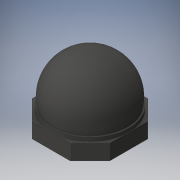
# Autodesk Inventor part: Drone Cover
Saved by Autodesk Inventor 2016 (Build 200138000, 138)
## iProperties
Created: 2015-05-23
Part Number: Drone Cover
Material: Generic
Document SubType Name: Modeling
Designer: Admin
Density: 1 g/cm^3
Appearance: Default
Mass: 29.2837 g
Surface Area: 921.431 cm^2
Volume: 29.2837 cm^3
Author: Admin
Autodesk Inventor part; units mm, degrees
ref_plane "YZ Plane" through (0, 0, 0) normal (1, 0, 0) x (0, 1, 0)
ref_plane "XY Plane" through (0, 0, 0) normal (0, 0, 1) x (1, 0, 0)
sketch "Sketch1" plane through (0, 0, 0) normal (0, 1, 0) x (-1, 0, 0)
  arc A0 (-63.5, 0) -> (63.5, 0) centre (0, 0) ccw
  line L0 (63.5, 0) -> (-63.5, 0)
  constraints: 2 end point, 2 point on circle, 1 centre point, 1 coincident, 1 horizontal
revolve "Revolution1" add sketch "Sketch1" angle 360 about axis through (-63.5, 0, 0) along (1, 0, 0)
ref_plane "Work Plane1" through (0, 12.7, 0) normal (0, 1, 0) x (-1, 0, 0)
sketch "Sketch2" plane through (0, 12.7, 0) normal (0, 1, 0) x (-1, 0, 0)
  circle A0 centre (0, 0) radius 63.5
  dimension "d3" = 127
  constraints: 1 centre point, 1 coincident
  measures "d3" diameter of A0
extrude "Extrusion1" cut sketch "Sketch2" along normal blind 50.8
sketch "Sketch3" plane through (0, 0, 0) normal (0, 0, 1) x (1, 0, 0)
  line L0 (-62.217, 12.7) -> (62.217, 12.7) projected
  line L1 (-62.217, 19.05) -> (62.217, 19.05)
  line L2 (0, 12.7) -> (0, 19.05)
  line L3 (-62.217, 12.7) -> (-63.2838, 12.7)
  line L4 (-63.2838, 19.05) -> (-62.217, 19.05)
  line L5 (62.217, 12.7) -> (63.2838, 12.7)
  line L6 (63.2838, 19.05) -> (62.217, 19.05)
  line L7 (63.2838, 12.7) -> (64.5792, 12.7)
  line L8 (64.5792, 12.7) -> (64.5792, 19.05)
  line L9 (64.5792, 19.05) -> (63.2838, 19.05)
  line L10 (-63.2838, 12.7) -> (-64.5792, 12.7)
  line L11 (-64.5792, 12.7) -> (-64.5792, 19.05)
  line L12 (-64.5792, 19.05) -> (-63.2838, 19.05)
  dimension "d6" = 6.35
  dimension "d33" = 1.0668
  dimension "d34" = 1.0668
  dimension "d36" = 1.2954
  dimension "d37" = 1.2954
  constraints: 24 end point, 4 perpendicular, 3 horizontal, 2 midpoint, 2 point on line
  measures "d6" distance of L0.start L1.start
  measures "d33" distance of L0.start L3.end
  measures "d34" distance of L0.end L5.end
  measures "d36" distance of L5.end L7.end
  measures "d37" distance of L3.end L10.end
ref_plane "Work Plane2" through (0, 19.05, 0) normal (0, 1, 0) x (1, 0, 0)
sketch "Sketch5" plane through (0, 19.05, 0) normal (0, 1, 0) x (1, 0, 0)
  line L0 (64.1257, 31.5673) -> (64.1257, -31.5673)
  line L1 (64.1257, -31.5673) -> (31.5673, -64.1257)
  line L2 (31.5673, -64.1257) -> (-31.5673, -64.1257)
  line L3 (-31.5673, -64.1257) -> (-64.1257, -31.5673)
  line L4 (-64.1257, -31.5673) -> (-64.1257, 31.5673)
  line L5 (-64.1257, 31.5673) -> (-31.5673, 64.1257)
  line L6 (-31.5673, 64.1257) -> (31.5673, 64.1257)
  line L7 (31.5673, 64.1257) -> (64.1257, 31.5673)
  point P0 (0, 0)
  point P1 (0, 0)
  constraints: 16 end point
extrude "Extrusion2" add sketch "Sketch5" along normal blind 25.4
revolve "Revolution3" add sketch "Sketch3" angle 360 about axis through (0, 12.7, 0) along (0, 1, 0)
shell "Shell2" thickness 0.6375 removed faces 1 at (-21.3752, 44.45, 10.5224)
move or copy body "Move Body1" bodies to move or copy 1 copy no rotation origin (0, 0, 0) rotation axis (-1, 0, 0) rotation angle -180 translate (0, 88.9, 128.2514)
body "Solid1"
